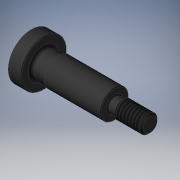
# Autodesk Inventor part: LMSBP4-10
Saved by Autodesk Inventor 2019 (Build 230136000, 136)
## iProperties
Created: 2024-03-18
Part Number: LMSBP4-10
Material: Generic
Catalog Web Link: www.cadenas.de
Description: LMSBP-Low Head Shoulder Bolts - Shaft Diameter Tolerance g6
Vendor: MISUMI
Document SubType Name: Modeling
Designer: psAdmin
Manufacturer: MISUMI
Mass: 0.199921 g
Surface Area: 2.7955 cm^2
Volume: 0.199921 cm^3
Density: 1 g/cm^3
Appearance: PSOLRGB-175-175-175
Category: PARTsolutions
Company: MISUMI
Title: LMSBP4-10
Author: Cadenas PARTsolutions
Comments: Low Head Shoulder Bolts - Shaft Diameter Tolerance g6
PSOL_IDENT_0: {$CADENAS_DATA/23d-libs/misumi/metric/27_screws_nuts/lmsbp.prj},176 {VTYP=3D},{NB=LMSBP4-10},{LINA=L
PSOL_IDENT_1: MSBP4-10},{NN=LMSBP},{DATE=15.07.2021 02:22:06},{GEOMDATE=29.06.2021 01:25:54},{VERSION=},{LINEID=10
PSOL_IDENT_2: },{WBVAR=ALT1,L,LC,FC},{WBNUMERIC=L,LC,FC}  {NB=LMSBP4-10},{LINA=LMSBP4-10},{KT=DUMMY},{PN=LMSBP4-10
PSOL_IDENT_3: },{TYPE=LMSBP},{SC=A2-90},{D=4.0},{DTOL=-0.004/-0.012},{ALT1=},{ALT1ALG= '' , 'w/o LC (Length (L))'
PSOL_IDENT_4: , 'LC' , 'with LC (Length (L))' },{L=10},{LALG=10,15,20,25,30},{LC=0.0},{F=5},{FC=0.0},{MP=2.5x0.45}
PSOL_IDENT_5: ,{A=6.5},{E=2.0},{B=2.5},{C=1.6},{N1=2.0},{D1=4.5},{N2=1.2},{D2=2.7},{M=2.5},{P=0.45},{LCALG=0},{LCM
PSOL_IDENT_6: AX=37.5},{FCALG=0},{FCMIN=2.5},{FCMAX=7.500},{EE=0.19},{FF=0.25}
NB: LMSBP4-10
NN: LMSBP
NT: Low Head Shoulder Bolts - Shaft Diameter Tolerance g6
NBSYN: $PN.
LINA: LMSBP4-10
CATALOG: Misumi
PN: LMSBP4-10
TYPE: LMSBP
SC: A2-90
D: 4
ALT1: w/o LC (Length (L))
L: 10
LC: 0
F: 5
FC: 0
MP: 2.5x0.45
A: 6.5
E: 2
B: 2.5
C: 1.6
N1: 2
D1: 4.5
N2: 1.2
D2: 2.7
SUPPLIER: MISUMI
ARTICLENO: LMSBP4-10
BOMINFO: LMSBP4-10
CREATOR: CADENAS GmbH
Autodesk Inventor part; units mm, degrees
ref_plane "YZ Plane" through (0, 0, 0) normal (1, 0, 0) x (0, 1, 0)
ref_plane "XZ Plane" through (0, 0, 0) normal (0, 1, 0) x (-1, 0, 0)
ref_plane "XY Plane" through (0, 0, 0) normal (0, 0, 1) x (1, 0, 0)
sketch "_____1" plane through (0, 0, 0) normal (0, 0, 1) x (1, 0, 0)
  line L0 (15, 0) -> (0.3217, 0)
  line L1 (0.3217, 0) -> (-0.4, 1.25)
  line L2 (-0.4, 1.25) -> (-2, 1.25)
  line L3 (-2, 1.25) -> (-2, 2.9036)
  line L4 (-2, 2.9036) -> (-1.8, 3.25)
  line L5 (-1.8, 3.25) -> (-0.1, 3.25)
  line L6 (-0.1, 3.25) -> (0, 3.15)
  line L7 (0, 3.15) -> (0, 2.25)
  arc A0 (0, 2.25) -> (0.44, 1.81) centre (0.44, 2.25) ccw
  line L8 (0.44, 1.81) -> (1.81, 1.81)
  line L9 (1.81, 1.81) -> (2, 2)
  line L10 (2, 2) -> (9.9, 2)
  line L11 (9.9, 2) -> (10, 1.9)
  line L12 (10, 1.9) -> (10, 1.2)
  arc A1 (10, 1.2) -> (10.2, 1) centre (10.2, 1.2) ccw
  line L13 (10.2, 1) -> (10.95, 1)
  line L14 (10.95, 1) -> (11.2, 1.25)
  line L15 (11.2, 1.25) -> (14.724, 1.25)
  line L16 (14.724, 1.25) -> (15, 0.974)
  line L17 (15, 0.974) -> (15, 0)
  line L18 (15, 0) -> (0.3217, 0)
  constraints: 38 end point, 4 point on circle, 2 centre point
revolve "Revolution1" add sketch "_____1" angle 360 about axis through (15, 0, 0) along (1, 0, 0)
thread "Thread1" size "M2.5x0.45" class "6g" standard "ISO Metric profile" full length
sketch "_____2" plane through (-2, 0, 0) normal (1, 0, 0) x (0, 0, -1)
  line L0 (-1.25, -0.7217) -> (0, -1.4434)
  line L1 (0, -1.4434) -> (1.25, -0.7217)
  line L2 (1.25, -0.7217) -> (1.25, 0.7217)
  line L3 (1.25, 0.7217) -> (0, 1.4434)
  line L4 (0, 1.4434) -> (-1.25, 0.7217)
  line L5 (-1.25, 0.7217) -> (-1.25, -0.7217)
  constraints: 12 end point
extrude "Extrusion1" cut sketch "_____2" along normal blind 1.6
body "Solid1"
